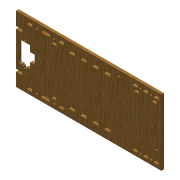
# Autodesk Inventor part: base
Saved by Autodesk Inventor 2016 (Build 200138000, 138)
## iProperties
Created: 2014-07-12
Part Number: base
Material: Plywood, Finish
Document SubType Name: Modeling
Designer: Sebastian
Density: 0.552 g/cm^3
Appearance: Plywood - New
Description: http://www.wickes.co.uk/Wickes-Non-Structural-Hardwood-Plywood-3-6x607x1829mm/p/110513
Mass: 18.9298 g
Surface Area: 263.847 cm^2
Volume: 34.2931 cm^3
Author: Sebastian
Autodesk Inventor part; units mm, degrees
ref_plane "YZ Plane" through (0, 0, 0) normal (1, 0, 0) x (0, 1, 0)
sketch "Base" plane through (0, 0, 0) normal (0, 1, 0) x (-1, 0, 0)
  line L0 (0, 0) -> (150, 0)
  line L1 (150, 0) -> (150, -75)
  line L2 (150, -75) -> (0, -75)
  line L3 (0, -75) -> (0, 0)
  dimension "d0" = 150
  dimension "d1" = 75
  constraints: 8 end point, 2 parallel, 1 horizontal, 1 perpendicular
  measures "d0" distance of L1.end L2.end
  measures "d1" distance of L0.end L1.end
extrude "Extrusion1" add sketch "Base" along normal blind 3
sketch "Sketch2" plane through (0, 3, 0) normal (0, 1, 0) x (1, 0, 0)
  line L0 (-3, 4) -> (-9, 4)
  line L1 (-9, 4) -> (-9, 7)
  line L2 (-9, 7) -> (-3, 7)
  line L3 (-3, 7) -> (-3, 4)
  line L4 (-150, 0) -> (0, 0) projected
  line L5 (0, 0) -> (0, 75) projected
  line L6 (-15, 4) -> (-21, 4)
  line L7 (-21, 4) -> (-21, 7)
  line L8 (-21, 7) -> (-15, 7)
  line L9 (-15, 7) -> (-15, 4)
  line L10 (-27, 7) -> (-33, 7)
  line L11 (-33, 7) -> (-33, 4)
  line L12 (-33, 4) -> (-27, 4)
  line L13 (-27, 4) -> (-27, 7)
  circle A0 centre (-24, 5.5) radius 1.5
  circle A1 centre (-12, 5.5) radius 1.5
  dimension "d4" = 6
  dimension "d5" = 3
  dimension "d6" = 4
  dimension "d7" = 3
  dimension "d100" = 6
  dimension "d101" = 6
  dimension "d102" = 6
  dimension "d103" = 6
  dimension "d104" = 3
  dimension "d107" = 3
  dimension "d108" = 3
  dimension "d109" = 3
  dimension "d110" = 3
  constraints: 24 end point, 6 parallel, 3 horizontal, 3 perpendicular, 2 centre point, 2 point on line
  measures "d4" distance of L1.end L2.end
  measures "d5" distance of L0.end L1.end
  measures "d6" distance between parallel lines of L0 L4
  measures "d7" distance between parallel lines of L5 L3
  measures "d100" distance of L7.end L8.end
  measures "d101" distance of L12.end L11.end
  measures "d102" distance between parallel lines of L13 L7
  measures "d103" distance between parallel lines of L1 L9
  measures "d104" distance of L10.end L11.end
  measures "d107" diameter of A0
  measures "d108" distance from line of A0.centre L13
  measures "d109" diameter of A1
  measures "d110" distance from line of L9 A1.centre
extrude "Extrusion2" cut sketch "Sketch2" against normal blind 4
ref_plane "Work Plane1" through (-75, 0, 0) normal (1, 0, 0) x (0, 0, -1)
ref_plane "Work Plane2" through (-150, 0, -37.5) normal (0, 0, 1) x (1, 0, 0)
mirror "Mirror3" about plane through (-150, 0, -37.5) normal (0, 0, 1) of "Extrusion2"
sketch "Sketch5" plane through (0, 3, 0) normal (0, 1, 0) x (1, 0, 0)
  line L0 (-56.1341, 6.5) -> (-3.1341, 6.5)
  line L1 (-3.1341, 6.5) -> (-3.1341, 71.5)
  line L2 (-3.1341, 71.5) -> (-56.1341, 71.5)
  line L3 (-56.1341, 71.5) -> (-56.1341, 6.5)
  line L4 (0, 75) -> (-150, 75) projected
  line L5 (-54.1341, 6.5) -> (-16.1341, 6.5)
  line L6 (-16.1341, 6.5) -> (-16.1341, 6.5)
  line L7 (-19.1341, 3.5) -> (-51.1341, 3.5)
  line L8 (-54.1341, 6.5) -> (-54.1341, 6.5)
  line L9 (-51.1341, 3.5) -> (-54.1341, 6.5)
  line L10 (-16.1341, 6.5) -> (-19.1341, 3.5)
  circle A0 centre (-5.6341, 56.5) radius 1.6
  circle A1 centre (-49.1341, 6) radius 1.6
  circle A2 centre (-21.6341, 6) radius 1.6
  point P0 (0, 0)
  point P1 (-16.1341, 3.5)
  point P2 (-54.1341, 3.5)
  dimension "d29" = 53
  dimension "d30" = 65
  dimension "d31" = 3.5
  dimension "d32" = 38
  dimension "d33" = 3
  dimension "d34" = 2
  dimension "d35" = 13
  dimension "d36" = 3
  dimension "d37" = 3
  dimension "d38" = 3
  dimension "d39" = 3
  dimension "d40" = 3.2
  dimension "d41" = 15
  dimension "d42" = 50.5
  dimension "d43" = 3.2
  dimension "d44" = 65.5
  dimension "d45" = 7
  dimension "d46" = 3.2
  constraints: 20 end point, 5 point on line, 4 parallel, 3 centre point, 2 horizontal, 2 perpendicular
  measures "d29" distance of L2.end L1.end
  measures "d30" distance of L1.end L0.end
  measures "d31" distance between parallel lines of L4 L2
  measures "d32" distance of point (-16.134, 3.5) point (-54.134, 3.5)
  measures "d33" distance of L5.end point (-16.134, 3.5)
  measures "d34" distance between parallel lines of L3 L8
  measures "d35" distance between parallel lines of L1 L6
  measures "d36" distance of L7.end point (-54.134, 3.5)
  measures "d37" distance of L8.start point (-54.134, 3.5)
  measures "d38" distance of L6.end point (-16.134, 3.5)
  measures "d39" distance of L7.start point (-16.134, 3.5)
  measures "d40" diameter of A0
  measures "d41" distance from line of A0.centre L2
  measures "d42" distance from line of L3 A0.centre
  measures "d43" diameter of A1
  measures "d44" distance from line of A1.centre L2
  measures "d45" distance from line of L3 A1.centre
  measures "d46" diameter of A2
extrude "Extrusion4" cut sketch "Sketch5" against normal blind 4 contours A1 L0 | L0 A1 | A0
sketch "Sketch6" plane through (0, 3, 0) normal (0, 1, 0) x (1, 0, 0)
  line L0 (-5.25, 9.5) -> (-10.75, 9.5)
  line L1 (-10.75, 9.5) -> (-10.75, 12)
  line L2 (-10.75, 12) -> (-5.25, 12)
  line L3 (-5.25, 12) -> (-5.25, 9.5)
  line L4 (-9, 7) -> (-3, 7) projected
  line L5 (-3, 7) -> (-3, 4) projected
  line L6 (-25.25, 9.5) -> (-30.75, 9.5)
  line L7 (-30.75, 9.5) -> (-30.75, 12)
  line L8 (-30.75, 12) -> (-25.25, 12)
  line L9 (-25.25, 12) -> (-25.25, 9.5)
  line L10 (-27, 7) -> (-33, 7) projected
  line L11 (-27, 4) -> (-27, 7) projected
  point P0 (0, 0)
  dimension "d49" = 5.5
  dimension "d50" = 2.5
  dimension "d51" = 2.5
  dimension "d52" = 2.25
  dimension "d53" = 5.5
  dimension "d54" = 2.5
  dimension "d105" = 2.5
  dimension "d106" = 1.75
  constraints: 16 end point, 4 parallel, 2 horizontal, 2 perpendicular
  measures "d49" distance of L1.end L2.end
  measures "d50" distance of L0.end L1.end
  measures "d51" distance between parallel lines of L4 L0
  measures "d52" distance between parallel lines of L3 L5
  measures "d53" distance of L7.end L8.end
  measures "d54" distance of L6.end L7.end
  measures "d105" distance between parallel lines of L6 L10
  measures "d106" distance between parallel lines of L9 L11
extrude "Extrusion5" cut sketch "Sketch6" against normal blind 4
sketch "Sketch7" plane through (0, 3, 0) normal (0, 1, 0) x (1, 0, 0)
  line L0 (-58, 8.5) -> (-65, 8.5)
  line L1 (-65, 8.5) -> (-65, 11.5)
  line L2 (-65, 11.5) -> (-58, 11.5)
  line L3 (-58, 11.5) -> (-58, 8.5)
  line L4 (0, 0) -> (0, 75) projected
  line L5 (-150, 0) -> (0, 0) projected
  dimension "d59" = 7
  dimension "d60" = 3
  dimension "d61" = 58
  dimension "d62" = 8.5
  constraints: 8 end point, 2 parallel, 1 horizontal, 1 perpendicular
  measures "d59" distance of L1.end L2.end
  measures "d60" distance of L0.end L1.end
  measures "d61" distance between parallel lines of L4 L3
  measures "d62" distance between parallel lines of L5 L0
extrude "Extrusion6" cut sketch "Sketch7" against normal blind 4
mirror "Mirror7" about plane through (-75, 0, 0) normal (1, 0, 0) of "Extrusion6"
sketch "Sketch8" plane through (0, 3, 0) normal (0, 1, 0) x (1, 0, 0)
  line L0 (-78.5, 8.338) -> (-71.5, 8.338)
  line L1 (-71.5, 8.338) -> (-71.5, 11.338)
  line L2 (-71.5, 11.338) -> (-78.5, 11.338)
  line L3 (-78.5, 11.338) -> (-78.5, 8.338)
  line L4 (-85, 11.5) -> (-85, 8.5) projected
  point P0 (0, 0)
  dimension "d65" = 7
  dimension "d66" = 3
  dimension "d67" = 6.5
  constraints: 8 end point, 2 parallel, 1 horizontal, 1 perpendicular
  measures "d65" distance of L2.end L1.end
  measures "d66" distance of L1.end L0.end
  measures "d67" distance between parallel lines of L3 L4
extrude "Extrusion7" cut sketch "Sketch8" against normal blind 4
mirror "Mirror8" about plane through (-150, 0, -37.5) normal (0, 0, 1) of "Extrusion6", "Mirror7", "Extrusion7"
sketch "Sketch9" plane through (-150, 0, -75) normal (-1, 0, 0) x (0, 0, 1)
  line L0 (0, 0) -> (75, 0)
  line L1 (75, 0) -> (75, 3)
  line L2 (75, 3) -> (0, 3)
  line L3 (0, 3) -> (0, 0)
  constraints: 8 end point, 2 parallel, 1 horizontal, 1 perpendicular
extrude "Extrusion8" add sketch "Sketch9" along normal blind 15
sketch "Sketch10" plane through (0, 0, 0) normal (0, -1, 0) x (1, 0, 0)
  line L0 (-162, -26) -> (-149, -26)
  line L1 (-162, -49.5) -> (-162, -26)
  line L2 (-165, -75) -> (-165, 0) projected
  line L3 (-165, -75) -> (0, -75) projected
  line L4 (0, 0) -> (-165, 0) projected
  line L5 (-149, -32.75) -> (-144, -32.75)
  line L6 (-144, -32.75) -> (-144, -42.75)
  line L7 (-144, -42.75) -> (-149, -42.75)
  line L8 (-149, -26) -> (-149, -32.75)
  line L9 (-149, -42.75) -> (-149, -49.5)
  circle A0 centre (-155.5, -24.2) radius 1.25
  arc A1 (-156.75, -51.3) -> (-154.25, -51.3) centre (-155.5, -51.3) ccw
  line L10 (-152.75, -49.5) -> (-152.75, -50.4)
  line L11 (-152.75, -50.4) -> (-154.25, -50.4)
  line L12 (-158.25, -49.5) -> (-158.25, -50.4)
  line L13 (-158.25, -50.4) -> (-156.75, -50.4)
  line L14 (-149, -49.5) -> (-152.75, -49.5)
  line L15 (-154.25, -50.4) -> (-154.25, -51.3)
  line L16 (-156.75, -51.3) -> (-156.75, -50.4)
  line L17 (-158.25, -49.5) -> (-162, -49.5)
  dimension "d74" = 3
  dimension "d75" = 75
  dimension "d76" = 26
  dimension "d83" = 13
  dimension "d84" = 13
  dimension "d85" = 5
  dimension "d86" = 10
  dimension "d89" = 6.75
  dimension "d117" = 2.5
  dimension "d118" = 6.5
  dimension "d119" = 1.8
  constraints: 30 end point, 7 perpendicular, 4 parallel, 2 centre point, 2 horizontal, 2 point on circle, 1 point on line, 1 vertical
  measures "d74" distance between parallel lines of L1 L2
  measures "d75" distance between parallel lines of L3 L4
  measures "d76" distance between parallel lines of L4 L0
  measures "d83" distance between parallel lines of L8 L1
  measures "d84" distance between parallel lines of L9 L1
  measures "d85" distance between parallel lines of L6 L8
  measures "d86" distance from line of L7 L5.end
  measures "d89" distance between parallel lines of L5 L0
  measures "d117" diameter of A0
  measures "d118" distance from line of L1 A0.centre
  measures "d119" distance from line of L0 A0.centre
extrude "Extrusion9" cut sketch "Sketch10" against normal blind 4
sketch "Sketch11" plane through (0, 0, 0) normal (0, -1, 0) x (1, 0, 0)
  line L0 (-127, -4) -> (-137, -4)
  line L1 (-146.9385, -7) -> (-152.9385, -7)
  line L2 (-152.9385, -7) -> (-152.9385, -4)
  line L3 (-152.9385, -4) -> (-146.9385, -4)
  line L4 (-146.9385, -4) -> (-146.9385, -7)
  line L5 (-111, -7) -> (-111, -4)
  line L6 (-111, -4) -> (-117, -4)
  line L7 (-165, -75) -> (-165, 0) projected
  line L8 (0, 0) -> (-165, 0) projected
  line L9 (-117, -4) -> (-117, -7)
  line L10 (-117, -7) -> (-111, -7)
  circle A0 centre (-142, -5.5) radius 1.5
  circle A1 centre (-122, -5.5) radius 1.5
  line L11 (-137, -4) -> (-127, -4)
  line L12 (-127, -4) -> (-127, -7)
  line L13 (-127, -7) -> (-137, -7)
  line L14 (-137, -7) -> (-137, -4)
  dimension "d91" = 6
  dimension "d92" = 3
  dimension "d93" = 6
  dimension "d96" = 12.0615
  dimension "d97" = 4
  dimension "d99" = 4
  dimension "d111" = 3
  dimension "d112" = 3
  dimension "d122" = 0
  dimension "d124" = 3
  dimension "d125" = 0
  dimension "d126" = 4
  dimension "d129" = 3
  constraints: 26 end point, 4 parallel, 3 perpendicular, 2 centre point, 2 horizontal, 1 point on line, 1 vertical
  measures "d91" distance of L2.end L3.end
  measures "d92" distance of L1.end L2.end
  measures "d93" distance of L6.end L5.end
  measures "d96" distance between parallel lines of L7 L2
  measures "d97" distance between parallel lines of L8 L3
  measures "d99" distance between parallel lines of L8 L6
  measures "d111" diameter of A0
  measures "d112" diameter of A1
  measures "d122" distance edge to line of A0 L1
  measures "d124" distance between parallel lines of L10 L6
  measures "d125" distance edge to line of A1 L10
  measures "d126" distance between parallel lines of L0 L8
  measures "d129" distance of L11.end L12.end
extrude "Extrusion10" cut sketch "Sketch11" against normal blind 4
mirror "Mirror9" about plane through (-150, 0, -37.5) normal (0, 0, 1) of "Extrusion10"
sketch "Sketch12" plane through (0, 0, 0) normal (0, -1, 0) x (1, 0, 0)
  line L0 (-165, 0) -> (-165, -75) projected
  line L1 (-165, -17.9) -> (-158, -17.9)
  line L2 (-158, -17.9) -> (-158, -15)
  line L3 (-158, -15) -> (-165, -15)
  line L4 (-165, -15) -> (-165, -17.9)
  line L5 (0, 0) -> (-165, 0) projected
  line L6 (-165, -57.1) -> (-158, -57.1)
  line L7 (-158, -57.1) -> (-158, -60)
  line L8 (-158, -60) -> (-165, -60)
  line L9 (-165, -60) -> (-165, -57.1)
  line L10 (-165, -75) -> (0, -75) projected
  dimension "d130" = 7
  dimension "d131" = 2.9
  dimension "d132" = 15
  dimension "d133" = 7
  dimension "d134" = 2.9
  dimension "d135" = 15
  constraints: 16 end point, 4 parallel, 2 horizontal, 2 perpendicular, 2 point on line
  measures "d130" distance of L3.end L2.end
  measures "d131" distance of L2.end L1.end
  measures "d132" distance between parallel lines of L3 L5
  measures "d133" distance of L7.end L8.end
  measures "d134" distance of L6.end L7.end
  measures "d135" distance between parallel lines of L10 L8
extrude "Extrusion11" cut sketch "Sketch12" against normal blind 10
sketch "Sketch13" plane through (0, 0, 0) normal (0, -1, 0) x (1, 0, 0)
  line L0 (-124.75, -9.5) -> (-119.25, -9.5)
  line L1 (-119.25, -9.5) -> (-119.25, -12)
  line L2 (-119.25, -12) -> (-124.75, -12)
  line L3 (-124.75, -12) -> (-124.75, -9.5)
  circle A0 centre (-122, -5.5) radius 1.5 projected
  line L4 (-111, -7) -> (-117, -7) projected
  point P0 (0, 0)
  dimension "d138" = 5.5
  dimension "d139" = 2.5
  dimension "d140" = 2.5
  dimension "d141" = 2.75
  constraints: 8 end point, 2 parallel, 1 horizontal, 1 perpendicular
  measures "d138" distance of L1.end L2.end
  measures "d139" distance of L0.end L1.end
  measures "d140" distance between parallel lines of L0 L4
  measures "d141" distance from line of A0.centre L1
extrude "Extrusion12" cut sketch "Sketch13" against normal blind 10 contours L0 L1 L2 L3
mirror "Mirror10" about plane through (-150, 0, -37.5) normal (0, 0, 1) of "Extrusion12"
sketch "Sketch14" plane through (0, 0, 0) normal (0, -1, 0) x (1, 0, 0)
  line L0 (-85, -11.5) -> (-92, -11.5) projected
  line L1 (-85, -8.5) -> (-85, -11.5) projected
  line L2 (-92, -8.5) -> (-85, -8.5) projected
  line L3 (-92, -11.5) -> (-92, -8.5) projected
  line L4 (-78.5, -11.338) -> (-78.5, -8.338) projected
  line L5 (-78.5, -8.338) -> (-71.5, -8.338) projected
  line L6 (-71.5, -11.338) -> (-78.5, -11.338) projected
  line L7 (-71.5, -8.338) -> (-71.5, -11.338) projected
  line L8 (-98.5, -8.5) -> (-105.5, -8.5)
  line L9 (-105.5, -8.5) -> (-105.5, -11.5)
  line L10 (-105.5, -11.5) -> (-98.5, -11.5)
  line L11 (-98.5, -11.5) -> (-98.5, -8.5)
  point P0 (0, 0)
  dimension "d144" = 7
  dimension "d145" = 7
  dimension "d146" = 6.5
  dimension "d147" = 6.5
  constraints: 8 end point, 2 parallel, 1 horizontal, 1 perpendicular
  measures "d144" distance between parallel lines of L1 L3
  measures "d145" distance between parallel lines of L9 L11
  measures "d146" distance between parallel lines of L4 L1
  measures "d147" distance between parallel lines of L3 L11
extrude "Extrusion13" cut sketch "Sketch14" against normal blind 10 contours L11 L10 L9 L8
mirror "Mirror11" about plane through (-150, 0, -37.5) normal (0, 0, 1) of "Extrusion13"
ref_plane "Work Plane3" through (-75, 0, 0) normal (1, 0, 0) x (0, 0, -1)
ref_plane "Work Plane4" through (-75, 0, -75) normal (-1, 0, 0) x (0, 0, 1)
ref_plane "Work Plane5" through (-75, 0, -75) normal (-1, 0, 0) x (0, 0, 1)
equation "\"d37\" = d36"
equation "\"d38\" = d36"
equation "\"d39\" = d38"
equation "\"d133\" = d130"
body "Solid1"
